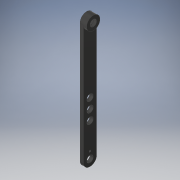
# Autodesk Inventor part: BT303_trajan20_21
Saved by Autodesk Inventor 2022.2 (Build 262287000, 287)
## iProperties
Company: HTBLA Kaindorf
RuleStatus: InUse
Created: 2022-09-09
Part Number: BT303_trajan20_21
Project: Zeichenmaschine_v2
Material: Kunststoff, undurchsichtig Schwarz
Description: gelenk b
Document SubType Name: Modeling
Designer: trajan20
Density: 0.952 g/cm^3
Appearance: Glatt - Schwarz
Mass: 17.9779 g
Surface Area: 105.378 cm^2
Volume: 18.8844 cm^3
AfterDocNew0: iProperties-Editor_aufrufen
Author: jan
Keywords: 2021
Autodesk Inventor part; units mm, degrees
ref_plane "YZ Plane" through (0, 0, 0) normal (1, 0, 0) x (0, 1, 0)
ref_plane "XZ Plane" through (0, 0, 0) normal (0, 1, 0) x (-1, 0, 0)
ref_plane "XY Plane" through (0, 0, 0) normal (0, 0, 1) x (1, 0, 0)
sketch "Skizze3" plane through (0, 0, 0) normal (0, 1, 0) x (-1, 0, 0)
  line L0 (0, 0) -> (0, -180) construction
  line L1 (-10, 0) -> (-10, -180)
  line L2 (10, -180) -> (10, 0)
  arc A0 (10, 0) -> (-10, 0) centre (0, 0) ccw
  arc A1 (-10, -180) -> (10, -180) centre (0, -180) ccw
  circle A2 centre (0, 0) radius 5
  circle A3 centre (0, -180) radius 5
  circle A4 centre (0, -170) radius 1.5
  circle A5 centre (0, -130) radius 5
  circle A6 centre (0, -115) radius 5
  circle A7 centre (0, -100) radius 5
  circle A8 centre (0, 0) radius 4.5
  point P0 (0, -90)
  dimension "d4" = 180
  dimension "d5" = 10
  dimension "d6" = 10
  dimension "d7" = 10
  dimension "d8" = 3
  dimension "d9" = 10
  dimension "d10" = 50
  dimension "d11" = 10
  dimension "d12" = 10
  dimension "d13" = 10
  dimension "d14" = 15
  dimension "d15" = 15
  dimension "d27" = 9
  constraints: 9 centre point, 8 end point, 4 point on circle, 4 point on line, 4 tangent, 3 coincident, 1 midpoint, 1 parallel, 1 vertical
  measures "d4" distance of L0.start L0.end
  measures "d5" radius of A0
  measures "d6" diameter of A2
  measures "d7" diameter of A3
  measures "d8" diameter of A4
  measures "d9" distance of L0.end A4.centre
  measures "d10" distance of L0.end A5.centre
  measures "d11" diameter of A5
  measures "d12" diameter of A6
  measures "d13" diameter of A7
  measures "d14" distance of A5.centre A6.centre
  measures "d15" distance of A6.centre A7.centre
  measures "d27" diameter of A8
extrude "Extrusion3" add sketch "Skizze3" along normal blind 5 contours A0 L2 A1 L1
sketch "Skizze4" plane through (0, 5, 0) normal (0, 1, 0) x (1, 0, 0)
  circle A0 centre (0, 0) radius 5 projected
  circle A1 centre (0, 0) radius 10
  dimension "d18" = 20
  constraints: 1 centre point, 1 coincident
  measures "d18" diameter of A1
extrude "Extrusion4" add sketch "Skizze4" along normal blind 5
extrude "Extrusion5" add sketch "Skizze3" along normal blind 6 contours A2
sketch "Skizze5" plane through (0, 0, 0) normal (0, -1, 0) x (1, 0, 0)
  circle A0 centre (0, -130) radius 5 projected
  circle A1 centre (0, -100) radius 5 projected
  circle A2 centre (0, -115) radius 5 projected
  circle A3 centre (0, -100) radius 4.5
  circle A4 centre (0, -115) radius 4.5
  circle A5 centre (0, -130) radius 4.5
  point P0 (0, 0)
  dimension "d28" = 9
  dimension "d29" = 9
  dimension "d30" = 9
  constraints: 3 centre point, 3 coincident
  measures "d28" diameter of A5
  measures "d29" diameter of A4
  measures "d30" diameter of A3
extrude "Extrusion7" add sketch "Skizze5" against normal blind 1
